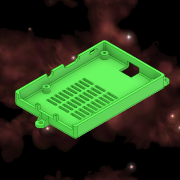
# Autodesk Inventor part: Bodem
Saved by Autodesk Inventor 2017 (Build 210142000, 142)
## iProperties
Created: 2016-12-17
Part Number: Bodem
Material: ABS Plastic
Document SubType Name: Modeling
Designer: bartv
Density: 1.06 g/cm^3
Appearance: Smooth - White
Author: bartv
## iProperties of the stored document Bodem_3DPrint.ipt
Created: 2016-12-19
Part Number: Bodem_3DPrint
Material: Generic
Document SubType Name: Modeling
Designer: bartv
Density: 1 g/cm^3
Appearance: Default
Author: bartv
Autodesk Inventor part; units mm, degrees
ref_plane "YZ Plane" through (0, 0, 0) normal (1, 0, 0) x (0, 1, 0)
ref_plane "XZ Plane" through (0, 0, 0) normal (0, 1, 0) x (-1, 0, 0)
ref_plane "XY Plane" through (0, 0, 0) normal (0, 0, 1) x (1, 0, 0)
sketch "Sketch3" plane through (0, 0, 0) normal (0, 1, 0) x (-1, 0, 0)
  line L0 (0, 0) -> (61, 0)
  line L1 (61, 0) -> (61, -90)
  line L2 (61, -90) -> (0, -90)
  line L3 (0, -90) -> (0, 0)
  dimension "d30" = 61
  dimension "d31" = 90
  constraints: 8 end point, 2 parallel, 1 horizontal, 1 perpendicular
  measures "d30" distance of L1.end L2.end
  measures "d31" distance between parallel lines of L0 L2
extrude "Extrusion2" add sketch "Sketch3" along normal blind 11.5
shell "Shell1" thickness 2 removed faces 1 at (-40.6667, 11.5, -60)
fillet "Fillet1" radius 2 8 edges at (-61, 5.75, 0) (0, 5.75, 0) (0, 5.75, -90) (-61, 5.75, -90) (-30.5, 0, -90) (-61, 0, -45) (-30.5, 0, 0) (0, 0, -45)
fillet "Fillet2" radius 1 8 edges at (-2, 2, -45) (-2, 6.75, -2) (-30.5, 2, -2) (-59, 2, -45) (-59, 6.75, -2) (-30.5, 2, -88) (-2, 6.75, -88) (-59, 6.75, -88)
sketch "Sketch4" plane through (-58, 2, -3) normal (0, 1, 0) x (1, 0, 0)
  line L0 (-1, 0) -> (-1, 84) projected
  arc A0 (0, 85) -> (-1, 84) centre (0, 84) ccw projected
  line L1 (0, 85) -> (55, 85) projected
  arc A1 (56, 84) -> (55, 85) centre (55, 84) ccw projected
  line L2 (56, 84) -> (56, 0) projected
  arc A2 (55, -1) -> (56, 0) centre (55, 0) ccw projected
  line L3 (55, -1) -> (0, -1) projected
  arc A3 (-1, 0) -> (0, -1) centre (0, 0) ccw projected
  arc A4 (-3, -1) -> (-1, -3) centre (-1, -1) ccw projected
  line L4 (-1, -3) -> (56, -3) projected
  arc A5 (56, -3) -> (58, -1) centre (56, -1) ccw projected
  line L5 (58, -1) -> (58, 85) projected
  arc A6 (58, 85) -> (56, 87) centre (56, 85) ccw projected
  line L6 (56, 87) -> (-1, 87) projected
  arc A7 (-1, 87) -> (-3, 85) centre (-1, 85) ccw projected
  line L7 (-3, 85) -> (-3, -1) projected
  circle A8 centre (52, 3) radius 3
  circle A9 centre (52, 61) radius 3
  circle A10 centre (3, 3) radius 3
  circle A11 centre (3, 61) radius 3
  point P0 (58, -3)
  dimension "d46" = 4
  dimension "d47" = 4
  dimension "d48" = 6
  dimension "d51" = 58
  dimension "d54" = 49
  constraints: 4 centre point, 4 coincident, 1 horizontal, 1 vertical, 9 other
  measures "d46" distance from line of L2 point (52, 3)
  measures "d47" distance from line of point (52, 3) L3
  measures "d48" diameter of A8
  measures "d51" distance of point (52, 3) point (52, 61)
  measures "d54" distance of point (52, 3) point (3, 3)
extrude "Extrusion3" add sketch "Sketch4" along normal blind 4 contours A8 | A9 | A10 | A11
hole "Hole1" at (-6, 6, -6) direction (0, -1, 0) diameter 2.013 depth 4 thread size "M2.5x0.45" class "6H" standard "ISO Metric profile"
pattern_linear "Rectangular Pattern1" count 2 spacing 49 along (-1, 0, 0) count 2 spacing 58 along (0, 0, -1) of "Hole1"
sketch "Sketch5" plane through (0, 2, -2) normal (1, 0, 0) x (0, 0, -1)
  line L0 (0, 0) -> (0, 9.5) projected
  line L1 (86, 0) -> (0, 0) projected
  line L2 (86, 9.5) -> (86, 0) projected
  line L3 (0, 9.5) -> (86, 9.5) projected
  line L4 (88, 9.5) -> (86, 9.5) projected
  line L5 (86, 9.5) -> (86, 0) projected
  line L6 (86, 0) -> (88, 0) projected
  line L7 (88, 0) -> (88, 9.5) projected
  circle A0 centre (54, 8.564) radius 3.05
  line L8 (0, -2) -> (86, -2) projected
  line L9 (27.5, 5.844) -> (37.5, 5.844)
  line L10 (37.5, 5.844) -> (38.85, 7.144)
  line L11 (38.85, 7.144) -> (40.1, 7.144)
  line L12 (40.1, 7.144) -> (40.1, 11.644)
  line L13 (40.1, 11.644) -> (24.9, 11.644)
  line L14 (24.9, 11.644) -> (24.9, 7.144)
  line L15 (24.9, 7.144) -> (26.15, 7.144)
  line L16 (26.15, 7.144) -> (27.5, 5.844)
  line L17 (7.3, 6.8) -> (14.9, 6.8) construction
  line L18 (8.8, 8.3) -> (13.4, 8.3)
  line L19 (13.4, 5.3) -> (8.8, 5.3)
  arc A1 (8.8, 8.3) -> (8.8, 5.3) centre (8.8, 6.8) ccw
  arc A2 (13.4, 5.3) -> (13.4, 8.3) centre (13.4, 6.8) ccw
  line L20 (-2, 9.5) -> (-2, 0) projected
  line L21 (7, 4) -> (1, 4) projected
  line L22 (4, 0) -> (1, 0) projected
  line L23 (1, 0) -> (4, 0) projected
  point P0 (-2, -2)
  point P1 (11.1, 6.8)
  dimension "d76" = 6.1
  dimension "d77" = 34
  dimension "d113" = 15.2
  dimension "d114" = 10
  dimension "d115" = 12.7
  dimension "d116" = 5.8
  dimension "d117" = 4.5
  dimension "d118" = 2.144
  dimension "d119" = 47.9
  dimension "d120" = 7.6
  dimension "d121" = 3
  dimension "d150" = 13.1
  dimension "d151" = 1.3
  dimension "d175" = 0.936
  constraints: 24 end point, 6 point on circle, 4 point on line, 4 tangent, 3 centre point, 2 equal length, 2 horizontal, 2 parallel, 2 perpendicular, 1 midpoint
  measures "d76" diameter of A0
  measures "d77" distance from line of L7 A0.centre
  measures "d113" distance of L12.end L13.end
  measures "d114" distance of L9.start L9.end
  measures "d115" distance of L10.end L15.end
  measures "d116" distance between parallel lines of L9 L13
  measures "d117" distance between parallel lines of L13 L11
  measures "d118" distance between parallel lines of L3 L13
  measures "d119" distance between parallel lines of L7 L12
  measures "d120" distance of L17.start L17.end
  measures "d121" distance between parallel lines of L19 L18
  measures "d150" distance from line of L20 point (11.1, 6.8)
  measures "d151" distance between parallel lines of L19 L21
  measures "d175" distance from line of L3 A0.centre
extrude "Extrusion4" cut sketch "Sketch5" against normal up to surface (2 mm away) contours L14 L13 L12 L3 | L3 L12 L11 L10 L9 L16 L15 L14 | A0 L3 | L3 A0 | L18 A2 L19 A1
sketch "Sketch7" plane through (-59, 2, 0) normal (0, 0, 1) x (1, 0, 0)
  line L0 (22.5, 3.5) -> (34.5, 3.5) construction
  line L1 (23.5, 4.5) -> (33.5, 4.5)
  arc A0 (23.5, 4.5) -> (22.5, 3.5) centre (23.5, 3.5) ccw
  arc A1 (34.5, 3.5) -> (33.5, 4.5) centre (33.5, 3.5) ccw
  line L2 (0, 0) -> (0, 9.5) projected
  line L3 (57, 0) -> (0, 0) projected
  line L4 (22.5, 3.5) -> (22.5, -2)
  line L5 (22.5, -2) -> (34.5, -2)
  line L6 (34.5, -2) -> (34.5, 3.5)
  line L7 (0, -2) -> (57, -2) projected
  point P0 (59, -2)
  point P1 (28.5, 3.5)
  dimension "d124" = 12
  dimension "d125" = 28.5
  dimension "d126" = 4.5
  dimension "d130" = 1
  dimension "d176" = 0
  constraints: 12 end point, 6 point on circle, 3 tangent, 2 centre point, 2 point on line, 1 horizontal, 1 midpoint, 1 parallel, 1 perpendicular, 1 vertical
  measures "d124" distance of L0.end L0.start
  measures "d125" distance from line of L2 point (28.5, 3.5)
  measures "d126" distance between parallel lines of L3 L1
  measures "d130" radius of A0
  measures "d176" distance between parallel lines of L5 L7
extrude "Extrusion6" cut sketch "Sketch7" against normal blind 10
sketch "Sketch8" plane through (-2, 11.5, -90) normal (0, 0, -1) x (-1, 0, 0)
  line L0 (2.4, -4.2) -> (18.8, -4.2)
  line L1 (18.8, -4.2) -> (18.8, 9.8)
  line L2 (18.8, 9.8) -> (2.4, 9.8)
  line L3 (2.4, 9.8) -> (2.4, -4.2)
  line L4 (0, 0) -> (57, 0) projected
  line L5 (-2, 0) -> (-2, -9.5) projected
  line L6 (21.7, -4.2) -> (37.2, -4.2)
  line L7 (37.2, -4.2) -> (37.2, 12)
  line L8 (37.2, 12) -> (21.7, 12)
  line L9 (21.7, 12) -> (21.7, -4.2)
  line L10 (7, -5.5) -> (1, -5.5) projected
  line L11 (7, -5.5) -> (1, -5.5) projected
  line L12 (1, -9.5) -> (7, -9.5) projected
  line L13 (40.1, -4.2) -> (55.6, -4.2)
  line L14 (55.6, -4.2) -> (55.6, 12)
  line L15 (55.6, 12) -> (40.1, 12)
  line L16 (40.1, 12) -> (40.1, -4.2)
  line L17 (0, -9.5) -> (0, 0) projected
  point P0 (-2, -11.5)
  dimension "d131" = 16.4
  dimension "d132" = 14
  dimension "d137" = 16.2
  dimension "d138" = 15.5
  dimension "d139" = 2.9
  dimension "d142" = 1.3
  dimension "d143" = 1.3
  dimension "d144" = 15.5
  dimension "d145" = 2.9
  dimension "d146" = 2.4
  dimension "d147" = 16.2
  dimension "d148" = 1.3
  constraints: 24 end point, 6 parallel, 3 horizontal, 3 perpendicular
  measures "d131" distance of L2.end L1.end
  measures "d132" distance between parallel lines of L0 L2
  measures "d137" distance between parallel lines of L6 L8
  measures "d138" distance between parallel lines of L7 L9
  measures "d139" distance between parallel lines of L1 L9
  measures "d142" distance between parallel lines of L0 L10
  measures "d143" distance between parallel lines of L10 L6
  measures "d144" distance of L15.end L14.end
  measures "d145" distance between parallel lines of L16 L7
  measures "d146" distance between parallel lines of L17 L3
  measures "d147" distance between parallel lines of L13 L15
  measures "d148" distance between parallel lines of L10 L13
extrude "Extrusion7" cut sketch "Sketch8" against normal up to surface (2 mm away)
sketch "Sketch9" plane through (0, 0, 0) normal (0, -1, 0) x (1, 0, 0)
  line L0 (-37.5, -71) -> (-47.5, -71) construction
  line L1 (-38.5, -70) -> (-46.5, -70)
  line L2 (-46.5, -72) -> (-38.5, -72)
  arc A0 (-38.5, -72) -> (-38.5, -70) centre (-38.5, -71) ccw
  arc A1 (-46.5, -70) -> (-46.5, -72) centre (-46.5, -71) ccw
  line L3 (-59, -88) -> (-59, -2) projected
  line L4 (-2, -88) -> (-59, -88) projected
  point P0 (0, 0)
  point P1 (-42.5, -71)
  dimension "d152" = 2
  dimension "d154" = 8
  dimension "d155" = 11.5
  dimension "d156" = 16
  constraints: 8 end point, 6 point on circle, 4 tangent, 2 centre point, 2 point on line, 1 horizontal, 1 midpoint, 1 parallel
  measures "d152" distance between parallel lines of L1 L2
  measures "d154" distance of A1.centre A0.centre
  measures "d155" distance from line of L3 L0.end
  measures "d156" distance between parallel lines of L4 L2
extrude "Extrusion8" cut sketch "Sketch9" against normal up to surface (2 mm away)
pattern_linear "Rectangular Pattern2" count 10 spacing 4 along (0, 0, 1) count 3 spacing 12 along (1, 0, 0) of "Extrusion8"
sketch "Sketch10" plane through (0, 0, 0) normal (0, -1, 0) x (1, 0, 0)
  line L0 (-59, -2) -> (-51, -2)
  line L1 (-51, -2) -> (-51, 4)
  line L2 (-59, 4) -> (-59, -2)
  line L3 (-10, -2) -> (-10, 4)
  line L4 (-34.5, -88) -> (-26.5, -88)
  line L5 (-26.5, -88) -> (-26.5, -94)
  line L6 (-34.5, -94) -> (-34.5, -88)
  line L7 (0, -88) -> (0, -2) projected
  line L8 (-59, -2) -> (-36.5, -2) projected
  line L9 (-2, -88) -> (-59, -88) projected
  arc A0 (-34.5, -94) -> (-26.5, -94) centre (-30.5, -94) ccw
  arc A1 (-51, 4) -> (-59, 4) centre (-55, 4) ccw
  arc A2 (-2, 4) -> (-10, 4) centre (-6, 4) ccw
  line L10 (-59, -88) -> (-59, -2) projected
  line L11 (-10, -2) -> (-2, -2)
  line L12 (-2, -2) -> (-2, 4)
  line L13 (-59, 0) -> (-2, 0) projected
  circle A3 centre (-6, 4) radius 1.5
  circle A4 centre (-55, 4) radius 1.5
  circle A5 centre (-30.5, -94) radius 1.5
  point P0 (0, 0)
  dimension "d177" = 8
  dimension "d181" = 8
  dimension "d183" = 26.5
  dimension "d184" = 8
  dimension "d185" = 8
  dimension "d190" = 4
  dimension "d191" = 6
  dimension "d192" = 4
  dimension "d194" = 6
  dimension "d197" = 0
  dimension "d202" = 8
  dimension "d203" = 4
  dimension "d204" = 6
  dimension "d205" = 2
  dimension "d206" = 2
  dimension "d207" = 4
  dimension "d208" = 3
  dimension "d209" = 3
  dimension "d210" = 3
  constraints: 18 end point, 6 centre point, 6 point on circle, 3 coincident, 3 horizontal, 3 perpendicular, 2 collinear, 2 parallel, 1 point on line
  measures "d177" distance between parallel lines of L2 L1
  measures "d181" distance between parallel lines of L5 L6
  measures "d183" distance between parallel lines of L7 L5
  measures "d184" diameter of A0
  measures "d185" diameter of A1
  measures "d190" distance from line of L1 A1.centre
  measures "d191" distance from line of L4 A0.centre
  measures "d192" distance from line of L6 A0.centre
  measures "d194" distance from line of L8 A1.centre
  measures "d197" distance between parallel lines of L10 L2
  measures "d202" distance between parallel lines of L3 L12
  measures "d203" radius of A2
  measures "d204" distance from line of L11 A2.centre
  measures "d205" distance between parallel lines of L7 L12
  measures "d206" distance between parallel lines of L13 L11
  measures "d207" distance from line of L3 A2.centre
  measures "d208" diameter of A3
  measures "d209" diameter of A4
  measures "d210" diameter of A5
extrude "Extrusion10" add sketch "Sketch10" against normal blind 2
sketch "Sketch11" plane through (-2, 0, 4) normal (1, 0, 0) x (0, 0, -1)
  line L0 (0, 2) -> (4, 2)
  line L1 (4, 2) -> (4, 7)
  line L2 (4, 7) -> (0, 2)
  line L3 (6, 0) -> (0, 0) projected
  line L4 (6, 2) -> (6, 11.5) projected
  point P0 (4, 0)
  dimension "d213" = 51.34
  dimension "d214" = 5
  dimension "d215" = 2
  dimension "d216" = 2
  constraints: 6 end point, 1 horizontal, 1 perpendicular
  measures "d213" angle of L0 L2
  measures "d214" distance of L0.end L1.end
  measures "d215" distance between parallel lines of L3 L0
  measures "d216" distance between parallel lines of L4 L1
extrude "Extrusion11" add sketch "Sketch11" against normal blind 1
pattern_linear "Rectangular Pattern3" count 2 spacing 7 along (-1, 0, 0) of "Extrusion11"
pattern_linear "Rectangular Pattern4" count 2 spacing 49 along (-1, 0, 0) of "Extrusion11", "Rectangular Pattern3"
sketch "Sketch12" plane through (-26.5, 0, -88) normal (1, 0, 0) x (0, 0, -1)
  line L0 (6, 2) -> (2, 2)
  line L1 (2, 2) -> (2, 7)
  line L2 (2, 7) -> (6, 2)
  line L3 (0, 0) -> (6, 0) projected
  point P0 (-88, 0)
  point P1 (0, 7.3)
  dimension "d225" = 5
  dimension "d226" = 2
  dimension "d227" = 2
  dimension "d228" = 51.34
  constraints: 6 end point, 1 horizontal, 1 perpendicular
  measures "d225" distance of L0.end L1.end
  measures "d226" distance between parallel lines of L3 L0
  measures "d227" distance from line of point (0, 7.3) L1
  measures "d228" angle of L0 L2
extrude "Extrusion12" add sketch "Sketch12" against normal blind 1
pattern_linear "Rectangular Pattern5" count 2 spacing 7 along (-1, 0, 0) of "Extrusion12"
sketch "Sketch13" plane through (0, 11.5, 0) normal (0, 1, 0) x (1, 0, 0)
  circle A0 centre (-22.3, 89) radius 0.8
  circle A1 centre (-40.7, 89) radius 0.8
  line L0 (-39.2, 88) -> (-39.2, 90) projected
  line L1 (-42.1, 88) -> (-39.2, 88) projected
  line L2 (-23.7, 88) -> (-20.8, 88) projected
  line L3 (-20.8, 88) -> (-20.8, 90) projected
  point P0 (0, 0)
  dimension "d234" = 1.6
  dimension "d235" = 1.6
  dimension "d236" = 1.5
  dimension "d237" = 1
  dimension "d238" = 1
  dimension "d239" = 1.5
  constraints: 2 centre point
  measures "d234" diameter of A0
  measures "d235" diameter of A1
  measures "d236" distance from line of L0 A1.centre
  measures "d237" distance from line of L1 A1.centre
  measures "d238" distance from line of L2 A0.centre
  measures "d239" distance from line of L3 A0.centre
extrude "Extrusion13" cut sketch "Sketch13" against normal blind 4
body "Solid2"
